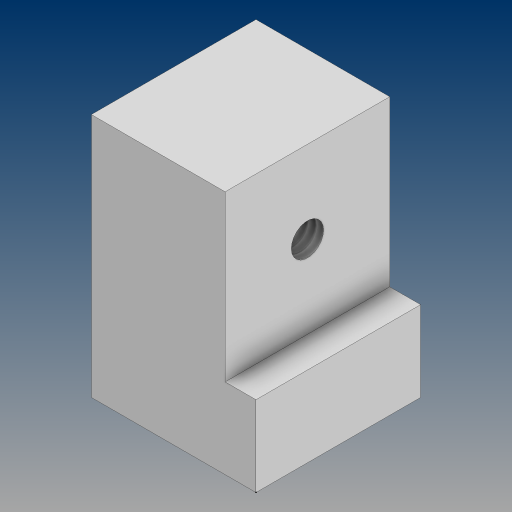
# Autodesk Inventor part: DragBarLinkage3 Billet
Saved by Autodesk Inventor 2024.3 (Build 283343000, 343)
## iProperties
Created: 2024-07-08
Part Number: DragBarLinkage3 Billet
Material: Generic
Document SubType Name: Modeling
Designer: Kenji
Density: 1 g/cm^3
Appearance: Default
Author: Kenji
Autodesk Inventor part; units mm, degrees
ref_plane "YZ Plane" through (0, 0, 0) normal (1, 0, 0) x (0, 1, 0)
ref_plane "XZ Plane" through (0, 0, 0) normal (0, 1, 0) x (-1, 0, 0)
ref_plane "XY Plane" through (0, 0, 0) normal (0, 0, 1) x (1, 0, 0)
sketch "Sketch1" plane through (0, 0, 0) normal (0, 1, 0) x (-1, 0, 0)
  line L0 (0, 0) -> (25.4, 0)
  line L1 (25.4, 0) -> (25.4, -25.4)
  line L2 (25.4, -25.4) -> (0, -25.4)
  line L3 (0, -25.4) -> (0, 0)
  dimension "d0" = 25.4
  dimension "d1" = 25.4
  constraints: 8 end point, 2 parallel, 1 horizontal, 1 perpendicular
  measures "d0" distance of L1.end L2.end
  measures "d1" distance of L0.end L1.end
extrude "Extrusion1" add sketch "Sketch1" along normal blind 37.7952
sketch "Sketch2" plane through (0, 0, 0) normal (0, -1, 0) x (1, 0, 0)
  line L0 (0, 0) -> (0, -25.4) projected
  line L1 (-25.4, 0) -> (0, 0) projected
  point P0 (-12.7, -12.7)
  point P1 (-12.7, 0)
  dimension "d4" = 12.7
  dimension "d5" = 12.7
  constraints: 1 midpoint
  measures "d4" distance from line of L0 point (-12.7, -12.7)
  measures "d5" distance of point (-12.7, 0) point (-12.7, -12.7)
hole "Hole1" at (-12.7, 0, -12.7) direction (0, 1, 0) diameter 4.9784 depth 19.05 thread size "1/4-20 UNC" class "2B" standard "ANSI Unified Screw Threads"
sketch "Sketch3" plane through (-25.4, 0, -25.4) normal (-1, 0, 0) x (0, 0, 1)
  line L0 (0, 37.7952) -> (25.4, 37.7952) projected
  line L1 (0, 0) -> (0, 37.7952) projected
  point P0 (25.4, 0)
  point P1 (12.7, 25.0952)
  dimension "d13" = 12.7
  dimension "d14" = 12.7
  measures "d13" distance from line of L0 point (12.7, 25.095)
  measures "d14" distance from line of L1 point (12.7, 25.095)
hole "Hole2" at (-25.4, 25.0952, -12.7) direction (1, 0, 0) diameter 4.9784 end through all thread size "1/4-20 UNC" class "2B" standard "ANSI Unified Screw Threads"
sketch "Sketch4" plane through (0, 37.7952, 0) normal (0, 1, 0) x (1, 0, 0)
  line L0 (0, 25.4) -> (-25.4, 25.4) projected
  line L1 (-25.4, 25.4) -> (-25.4, 0) projected
  line L2 (-25.4, 0) -> (0, 0) projected
  line L3 (0, 0) -> (0, 25.4) projected
  line L4 (-4.7625, 25.4) -> (-4.7625, 0)
  line L5 (-25.4, 0) -> (0, 0) projected
  dimension "d22" = 4.7625
  constraints: 2 end point, 2 point on line, 1 perpendicular
  measures "d22" distance between parallel lines of L3 L4
extrude "Extrusion2" cut sketch "Sketch4" against normal blind 25.4
extrude "Extrusion3" add sketch "Sketch4" against normal blind 25.4 contours L4 L2 L1 L0
sketch "Sketch6" plane through (-4.7625, 37.7952, 0) normal (1, 0, 0) x (0, 0, -1)
  line L0 (0, 0) -> (25.4, 0) projected
  line L1 (0, 0) -> (0, -25.4) projected
  point P0 (0, -37.7952)
  point P1 (12.7, -12.7)
  point P2 (12.7, 0)
  point P3 (0, -12.7)
  dimension "d28" = 12.7
  dimension "d29" = 12.7
  constraints: 2 midpoint
  measures "d28" distance of point (12.7, 0) point (12.7, -12.7)
  measures "d29" distance of point (0, -12.7) point (12.7, -12.7)
hole "Hole3" at (-4.7625, 25.0952, -12.7) direction (-1, 0, 0) diameter 4.9784 end through all thread size "1/4-20 UNC" class "2B" standard "ANSI Unified Screw Threads"
sketch "Sketch7" plane through (0, 0, 0) normal (0, -1, 0) x (1, 0, 0)
  point P0 (0, 0)
body "Solid1"
